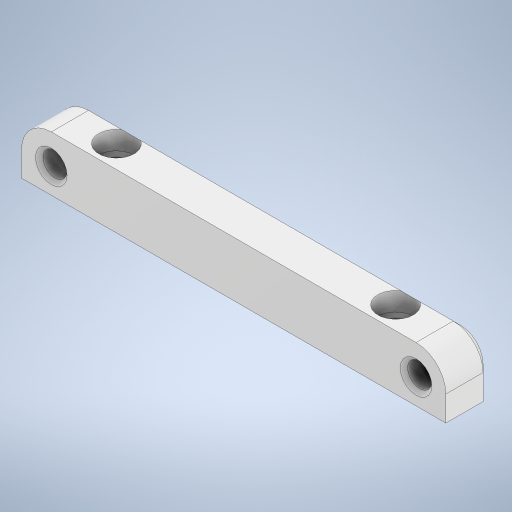
# Autodesk Inventor part: Front Panel Mount
Saved by Autodesk Inventor 2024 (Build 280153000, 153)
## iProperties
Created: 2024-12-02
Part Number: Front Panel Mount
Material: ABS Plastic
Document SubType Name: Modeling
Designer: Ishaan
Density: 1.06 g/cm^3
Appearance: Smooth - White
Author: Ishaan
Autodesk Inventor part; units mm, degrees
ref_plane "YZ Plane" through (0, 0, 0) normal (1, 0, 0) x (0, 1, 0)
ref_plane "XZ Plane" through (0, 0, 0) normal (0, 1, 0) x (-1, 0, 0)
ref_plane "XY Plane" through (0, 0, 0) normal (0, 0, 1) x (1, 0, 0)
sketch "Sketch1" plane through (0, 0, 0) normal (0, 0, 1) x (1, 0, 0)
  line L0 (-49, 0) -> (49, 0) construction
  line L1 (-53.7631, 0) -> (-51.3816, 4.125)
  line L2 (-51.3816, 4.125) -> (-46.6184, 4.125)
  line L3 (-46.6184, 4.125) -> (-44.2369, 0)
  line L4 (-44.2369, 0) -> (-46.6184, -4.125)
  line L5 (-46.6184, -4.125) -> (-51.3816, -4.125)
  line L6 (-51.3816, -4.125) -> (-53.7631, 0)
  line L7 (53.7631, 0) -> (51.3816, -4.125)
  line L8 (51.3816, -4.125) -> (46.6184, -4.125)
  line L9 (46.6184, -4.125) -> (44.2369, 0)
  line L10 (44.2369, 0) -> (46.6184, 4.125)
  line L11 (46.6184, 4.125) -> (51.3816, 4.125)
  line L12 (51.3816, 4.125) -> (53.7631, 0)
  line L13 (57, -8) -> (-57, -8)
  line L14 (-57, -8) -> (-57, 8)
  line L15 (-57, 8) -> (57, 8)
  line L16 (57, 8) -> (57, -8)
  line L17 (57, -8) -> (-57, 8) construction
  line L18 (-57, -8) -> (57, 8) construction
  line L19 (-57, -6.75) -> (57, -6.75)
  circle A0 centre (-49, 0) radius 8
  circle A1 centre (49, 0) radius 8
  point P0 (0, 0)
  point P1 (0, 0)
  point P2 (49, 8)
  point P3 (-49, 8)
  point P4 (-57, 0)
  point P5 (57, 0)
  dimension "d0" = 98
  dimension "d1" = 8.25
  dimension "d2" = 16
  dimension "d3" = 8
  dimension "d4" = 8
  dimension "d34" = 6.75
  constraints: 40 end point, 7 coincident, 3 horizontal, 3 midpoint, 3 point on line, 3 tangent, 2 centre point, 2 parallel, 2 perpendicular, 1 collinear, 26 other
  measures "d0" distance of L0.start L0.end
  measures "d1" distance between parallel lines of L5 L2
  measures "d2" distance of L13.end L14.end
  measures "d3" distance from line of L15 L0.start
  measures "d4" distance from line of point (-49, 0) L14
  measures "d34" distance from line of L19 L0.end
extrude "Extrusion1" add sketch "Sketch1" against normal blind 12 contours L1 L2 L3 L4 L5 L6 | L7 L8 L9 L10 L11 L12 | L19 A1 L16 | A1 L19 | L19 A0 L15 A1 | A0 L19 | L19 L14 A0 picked at (48.2061, -5.875) picked at (-49.7939, -5.875)
chamfer "Chamfer2" distance 2 angle 45 5 edges at (0, 8, -12) (54.6569, 5.6569, -12) (57, -3.375, -12) (-54.6569, 5.6569, -12) (-57, -3.375, -12)
sketch "Sketch2" plane through (-49, 8, 0) normal (0, 1, 0) x (1, 0, 0)
  line L0 (11.5, 6) -> (86.5, 6) construction
  line L1 (98, 0) -> (0, 0) projected
  line L2 (98, 12) -> (0, 12) projected
  line L3 (49, 0) -> (49, 12) construction
  point P0 (49, 6)
  dimension "d14" = 75
  constraints: 4 end point, 4 midpoint, 2 coincident, 1 horizontal
  measures "d14" distance of L0.start L0.end
hole "Hole1" at (-37.5, 8, -6) at (37.5, 8, -6) direction (0, -1, 0) diameter 5.4 end through all counterbore diameter 9.5 counterbore depth 5
sketch "Sketch3" plane through (0, 0, 0) normal (0, 0, 1) x (1, 0, 0)
  line L0 (-57, -6.75) -> (57, -6.75) projected
  arc A0 (-49, 8) -> (-57, 0) centre (-49, 0) ccw projected
  line L1 (-57, 0) -> (-57, -6.75) projected
  line L2 (57, -6.75) -> (57, 0) projected
  arc A1 (57, 0) -> (49, 8) centre (49, 0) ccw projected
  line L3 (49, 8) -> (-49, 8) projected
  point P0 (0, 0)
hole "Hole2" at (-49, 0, 0) at (49, 0, 0) direction (0, 0, -1) diameter 6.5 end through all
chamfer "Chamfer3" distance 1 angle 45 2 edges at (-49, 3.25, 0) (49, 3.25, 0)
equation "\"d4\" = d3"
body "Solid1"
